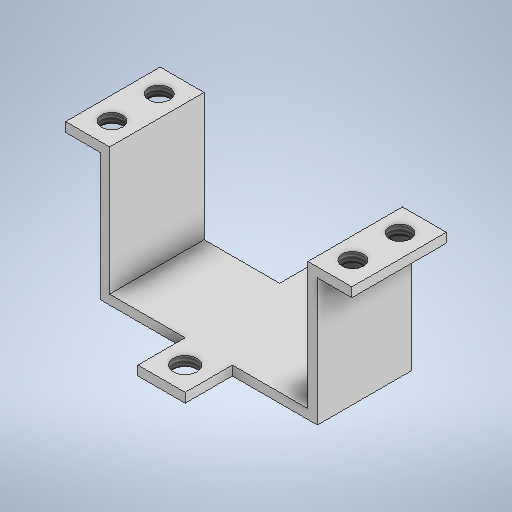
# Autodesk Inventor part: Servo Mount
Saved by Autodesk Inventor 2025.3 (Build 293356000, 356)
## iProperties
Created: 2026-04-10
Part Number: Servo Mount
Material: Generic
Document SubType Name: Modeling
Designer: abdul
Density: 1 g/cm^3
Appearance: Default
Author: abdul
Autodesk Inventor part; units mm, degrees
ref_plane "YZ Plane" through (0, 0, 0) normal (1, 0, 0) x (0, 1, 0)
ref_plane "XZ Plane" through (0, 0, 0) normal (0, 1, 0) x (-1, 0, 0)
ref_plane "XY Plane" through (0, 0, 0) normal (0, 0, 1) x (1, 0, 0)
sketch "Sketch1" plane through (0, 0, 0) normal (0, 0, 1) x (1, 0, 0)
  line L0 (2, 0) -> (44, 0)
  line L1 (46, 0) -> (46, -2)
  line L2 (46, -2) -> (0, -2)
  line L3 (0, -2) -> (0, 0)
  line L4 (46, 0) -> (46, 25)
  line L5 (53.3, 27) -> (53.3, 25)
  line L6 (53.3, 25) -> (46, 25)
  line L7 (23, -2) -> (23, 38) construction
  line L8 (0, 0) -> (0, 25)
  line L9 (-7.3, 27) -> (-7.3, 25)
  line L10 (-7.3, 25) -> (0, 25)
  line L11 (2, 0) -> (2, 27)
  line L12 (44, 0) -> (44, 27)
  line L13 (44, 27) -> (53.3, 27)
  line L14 (-7.3, 27) -> (2, 27)
  line L15 (18, -2) -> (18, 0)
  line L16 (28, -2) -> (28, 0)
  dimension "d0" = 46
  dimension "d4" = 2
  dimension "d5" = 40
  dimension "d8" = 2
  dimension "d9" = 27
  dimension "d11" = 9.3
  dimension "d20" = 2
  dimension "d29" = 5
  dimension "d30" = 10
  constraints: 34 end point, 7 vertical, 6 perpendicular, 3 symmetric about line, 2 horizontal, 2 point on line, 1 midpoint, 1 parallel
  measures "d0" distance of L1.end L2.end
  measures "d4" distance from line of L3.end L2
  measures "d5" distance of L7.start L7.end
  measures "d8" distance from line of L1.start L12
  measures "d9" distance of L0.start L11.end
  measures "d11" distance of L5.start L12.end
  measures "d20" distance of L5.start L5.end
  measures "d29" distance between parallel lines of L7 L15
  measures "d30" distance between parallel lines of L16 L15
extrude "Extrusion1" add sketch "Sketch1" along normal mid plane 20 contours L0 L15 L2 L3 L8 L10 L9 L14 L11 | L0 L12 L13 L5 L6 L4 L1 L2 L16
sketch "Sketch3" plane through (-7.3, 27, -10) normal (0, 1, 0) x (1, 0, 0)
  circle A0 centre (4.8, -5) radius 2.25
  line L0 (9.3, 0) -> (9.3, -20) projected
  line L1 (0, 0) -> (9.3, 0) projected
  circle A1 centre (4.8, -15) radius 2.25
  line L2 (7.3, -20) -> (53.3, -20) construction
  line L3 (30.3, -20) -> (30.3, 0) construction
  circle A2 centre (55.8, -5) radius 2.25
  circle A3 centre (55.8, -15) radius 2.25
  dimension "d21" = 4.5
  dimension "d22" = 4.5
  dimension "d23" = 5
  dimension "d24" = 4.5
  dimension "d25" = 10
  dimension "d26" = 4.5
  constraints: 4 centre point, 2 end point, 2 symmetric about line, 1 midpoint, 1 vertical, 2 other
  measures "d21" diameter of A0
  measures "d22" distance from line of L0 A0.centre
  measures "d23" distance from line of L1 A0.centre
  measures "d24" diameter of A1
  measures "d25" distance of A1.centre A0.centre
  measures "d26" distance from line of L0 A1.centre
extrude "Extrusion2" cut sketch "Sketch3" against normal through all
extrude "Extrusion3" add sketch "Sketch1" along normal mid plane 40 contours L0 L16 L2 L15
sketch "Sketch4" plane through (2, 0, 10) normal (0, 1, 0) x (1, 0, 0)
  circle A0 centre (21, -5) radius 2.5
  circle A1 centre (21, 25) radius 2.5
  line L0 (16, 30) -> (26, 30) projected
  line L1 (26, 20) -> (26, 30) projected
  line L2 (26, -10) -> (26, 0) projected
  line L3 (26, -10) -> (16, -10) projected
  point P0 (-2, 10)
  dimension "d33" = 5
  dimension "d34" = 5
  dimension "d35" = 5
  dimension "d36" = 5
  dimension "d37" = 5
  constraints: 2 centre point, 1 equal radius
  measures "d33" distance from line of L0 A1.centre
  measures "d34" distance from line of A1.centre L1
  measures "d35" diameter of A0
  measures "d36" distance from line of L2 A0.centre
  measures "d37" distance from line of L3 A0.centre
extrude "Extrusion4" cut sketch "Sketch4" against normal blind 5
thread "Thread1" size "M5x0.8" class "6H" standard "ANSI Metric M Profile" length 77
thread "Thread2" size "M4.5x0.75" class "6H" standard "ANSI Metric M Profile" length 77
thread "Thread3" size "M4.5x0.75" class "6H" standard "ANSI Metric M Profile" length 77
thread "Thread4" size "M4.5x0.75" class "6H" standard "ANSI Metric M Profile" length 77
thread "Thread5" size "M4.5x0.75" class "6H" standard "ANSI Metric M Profile" length 77
thread "Thread6" size "M5x0.8" class "6H" standard "ANSI Metric M Profile" length 77
equation "\"d11\" = d10"
equation "\"d26\" = d22"
equation "\"d36\" = d34"
equation "\"d37\" = d33"
equation "\"d38\" = d37"
equation "\"d10\" = 9.3"
body "Solid1"
